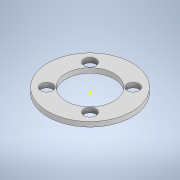
# Autodesk Inventor part: Pièce_moteur_maintient_test_1
Saved by Autodesk Inventor 2020.1 (Build 241239000, 239)
## iProperties
Created: 2019-07-26
Part Number: Pièce_moteur_maintient_test_1
Material: Générique
Document SubType Name: Modeling
Designer: marlo
Density: 1 g/cm^3
Appearance: Par défaut
Author: marlo
Autodesk Inventor part; units mm, degrees
ref_plane "YZ Plane" through (0, 0, 0) normal (1, 0, 0) x (0, 1, 0)
ref_plane "XZ Plane" through (0, 0, 0) normal (0, 1, 0) x (-1, 0, 0)
ref_plane "XY Plane" through (0, 0, 0) normal (0, 0, 1) x (1, 0, 0)
sketch "Esquisse1" plane through (0, 0, 0) normal (0, 1, 0) x (-1, 0, 0)
  point P0 (0, 0)
sketch "Esquisse2" plane through (0, 0, 0) normal (0, 1, 0) x (-1, 0, 0)
  point P0 (0, 0)
sketch "Esquisse3" plane through (0, 0, 0) normal (0, 1, 0) x (-1, 0, 0)
  line L0 (-6.5, 6.5) -> (6.5, 6.5) construction
  line L1 (6.5, 6.5) -> (6.5, -6.5) construction
  line L2 (6.5, -6.5) -> (-6.5, -6.5) construction
  line L3 (-6.5, -6.5) -> (-6.5, 6.5) construction
  line L4 (-6.5, 6.5) -> (6.5, -6.5) construction
  line L5 (6.5, 6.5) -> (-6.5, -6.5) construction
  line L6 (-11.5, 11.5) -> (11.5, 11.5) construction
  line L7 (11.5, 11.5) -> (11.5, -11.5) construction
  line L8 (11.5, -11.5) -> (-11.5, -11.5) construction
  line L9 (-11.5, -11.5) -> (-11.5, 11.5) construction
  line L10 (-11.5, 11.5) -> (11.5, -11.5) construction
  line L11 (11.5, 11.5) -> (-11.5, -11.5) construction
  line L12 (-6.5, 6.5) -> (-11.5, 6.5) construction
  line L13 (-11.5, 6.5) -> (-11.5, 11.5) construction
  line L14 (-11.5, 11.5) -> (-6.5, 11.5) construction
  line L15 (-6.5, 11.5) -> (-6.5, 6.5) construction
  line L16 (-6.5, -6.5) -> (-11.5, -6.5) construction
  line L17 (-11.5, -6.5) -> (-11.5, -11.5) construction
  line L18 (-11.5, -11.5) -> (-6.5, -11.5) construction
  line L19 (-6.5, -11.5) -> (-6.5, -6.5) construction
  line L20 (6.5, -6.5) -> (11.5, -6.5) construction
  line L21 (11.5, -6.5) -> (11.5, -11.5) construction
  line L22 (11.5, -11.5) -> (6.5, -11.5) construction
  line L23 (6.5, -11.5) -> (6.5, -6.5) construction
  line L24 (11.5, 11.5) -> (6.5, 11.5) construction
  line L25 (6.5, 11.5) -> (6.5, 6.5) construction
  line L26 (6.5, 6.5) -> (11.5, 6.5) construction
  line L27 (11.5, 6.5) -> (11.5, 11.5) construction
  circle A0 centre (9, 9) radius 2.5
  circle A1 centre (9, -9) radius 2.5
  circle A2 centre (-9, -9) radius 2.5
  circle A3 centre (-9, 9) radius 2.5
  circle A4 centre (0, 0) radius 17.5
  circle A5 centre (0, 0) radius 9.9893
  dimension "d1" = 13
  dimension "d2" = 13
  dimension "d3" = 5
  dimension "d4" = 35
  constraints: 56 end point, 12 parallel, 12 tangent, 6 centre point, 6 horizontal, 6 perpendicular, 2 coincident, 2 midpoint, 1 point on line
  measures "d1" distance of L0.end L1.end
  measures "d2" distance of L0.start L0.end
  measures "d3" distance between parallel lines of L2 L8
  measures "d4" diameter of A4
extrude "Extrusion1" add sketch "Esquisse3" along normal blind 2
